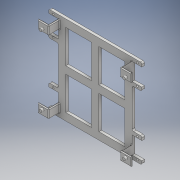
# Autodesk Inventor part: kadlub
Saved by Autodesk Inventor 2018 (Build 220112000, 112)
## iProperties
Created: 2020-10-03
Part Number: kadlub
Material: Ogólny
Document SubType Name: Modeling
Designer: Raven
Density: 1 g/cm^3
Appearance: Domyślna
Author: Raven
Autodesk Inventor part; units mm, degrees
ref_plane "YZ Plane" through (0, 0, 0) normal (1, 0, 0) x (0, 1, 0)
ref_plane "XZ Plane" through (0, 0, 0) normal (0, 1, 0) x (-1, 0, 0)
ref_plane "XY Plane" through (0, 0, 0) normal (0, 0, 1) x (1, 0, 0)
sketch "Szkic1" plane through (0, 0, 0) normal (0, 1, 0) x (-1, 0, 0)
  line L0 (0, 0) -> (50, 0) construction
  line L1 (50, 0) -> (50, -60) construction
  line L2 (50, -60) -> (0, -60) construction
  line L3 (0, -60) -> (0, 0) construction
  line L4 (50, -60) -> (20, -60) construction
  line L5 (20, -60) -> (20, -30) construction
  line L6 (20, -30) -> (50, -30) construction
  line L7 (50, -30) -> (50, -60) construction
  line L8 (20, -30) -> (76.5685, -86.5685) construction
  line L9 (20, -30) -> (100, -30) construction
  line L10 (50, -60) -> (-50, -60)
  line L11 (-50, -60) -> (-50, 60)
  line L12 (-50, 60) -> (50, 60)
  line L13 (50, 60) -> (50, -60)
  dimension "d0" = 50
  dimension "d1" = 60
  dimension "d2" = 30
  dimension "d3" = 30
  dimension "d4" = 80
  dimension "d5" = 45
  dimension "d6" = 100
  dimension "d7" = 120
  constraints: 28 end point, 6 parallel, 4 horizontal, 3 perpendicular, 1 equal length
  measures "d0" distance of L1.end L2.end
  measures "d1" distance of L0.end L1.end
  measures "d2" distance of L5.end L6.end
  measures "d3" distance of L4.end L5.end
  measures "d4" distance of L5.end L8.end
  measures "d5" angle of L8 L9
  measures "d6" distance of L11.end L12.end
  measures "d7" distance of L10.end L11.end
extrude "Wyciągnięcie proste1" add sketch "Szkic1" along normal blind 3.5
sketch "Szkic2" plane through (0, 0, 0) normal (0, -1, 0) x (1, 0, 0)
  line L0 (-50, 60) -> (-50, -60) construction
  line L1 (50, -60) -> (-50, -60) projected
  line L2 (-50, -60) -> (-63.2, -60)
  line L3 (-63.2, -60) -> (-63.2, -55)
  line L4 (-63.2, -55) -> (-50, -55)
  line L5 (-50, -55) -> (-50, -60)
  line L6 (-57.1, -55) -> (-57.1, -56.9) construction
  circle A0 centre (-57.1, -56.9) radius 1.25
  line L7 (-50, -55) -> (-50, -43.2) construction
  line L8 (-50, -60) -> (-50, 60) construction
  line L9 (-50, -43.2) -> (-68.7012, -43.2) construction
  line L10 (-50, -26.4) -> (-63.2, -26.4)
  line L11 (-63.2, -26.4) -> (-63.2, -31.4)
  line L12 (-63.2, -31.4) -> (-50, -31.4)
  line L13 (-50, -31.4) -> (-50, -26.4)
  line L14 (-57.1, -31.4) -> (-57.1, -29.5) construction
  circle A1 centre (-57.1, -29.5) radius 1.25
  line L15 (0, 0) -> (-82.4094, 0) construction
  line L16 (0, -60) -> (0, 60) construction
  line L17 (-50, -60) -> (-50, 60) construction
  line L18 (50, 60) -> (-50, 60)
  line L19 (-50, 60) -> (-63.2, 60)
  line L20 (-63.2, 60) -> (-63.2, 55)
  line L21 (-63.2, 55) -> (-50, 55)
  line L22 (-50, 55) -> (-50, 60)
  line L23 (-57.1, 55) -> (-57.1, 56.9) construction
  circle A2 centre (-57.1, 56.9) radius 1.25
  line L24 (-50, 55) -> (-50, 43.2) construction
  line L25 (-50, 60) -> (-50, -60) construction
  line L26 (-50, 43.2) -> (-68.7012, 43.2) construction
  line L27 (-63.2, 31.4) -> (-50, 31.4)
  line L28 (-50, 26.4) -> (-63.2, 26.4)
  line L29 (-63.2, 26.4) -> (-63.2, 31.4)
  line L30 (-57.1, 31.4) -> (-57.1, 29.5) construction
  circle A3 centre (-57.1, 29.5) radius 1.25
  line L31 (-50, 31.4) -> (-50, 26.4)
  line L32 (50, 60) -> (50, -60) construction
  line L33 (-50, -60) -> (50, -60)
  line L34 (50, -60) -> (63.2, -60)
  line L35 (63.2, -60) -> (63.2, -55)
  line L36 (63.2, -55) -> (50, -55)
  line L37 (50, -55) -> (50, -60)
  line L38 (57.1, -55) -> (57.1, -56.9) construction
  circle A4 centre (57.1, -56.9) radius 1.25
  line L39 (50, -55) -> (50, -43.2) construction
  line L40 (50, -60) -> (50, 60) construction
  line L41 (50, -43.2) -> (68.7012, -43.2) construction
  line L42 (63.2, -31.4) -> (50, -31.4)
  line L43 (50, -26.4) -> (63.2, -26.4)
  line L44 (63.2, -26.4) -> (63.2, -31.4)
  line L45 (57.1, -31.4) -> (57.1, -29.5) construction
  circle A5 centre (57.1, -29.5) radius 1.25
  line L46 (50, -31.4) -> (50, -26.4)
  line L47 (0, 0) -> (82.4094, 0) construction
  line L48 (63.2, 31.4) -> (50, 31.4)
  line L49 (57.1, 31.4) -> (57.1, 29.5) construction
  circle A6 centre (57.1, 29.5) radius 1.25
  line L50 (63.2, 26.4) -> (63.2, 31.4)
  line L51 (50, 31.4) -> (50, 26.4)
  line L52 (50, 26.4) -> (63.2, 26.4)
  line L53 (50, -60) -> (50, 60) construction
  line L54 (50, 60) -> (50, -60) construction
  line L55 (50, 43.2) -> (68.7012, 43.2) construction
  line L56 (63.2, 55) -> (50, 55)
  line L57 (50, 55) -> (50, 43.2) construction
  line L58 (57.1, 55) -> (57.1, 56.9) construction
  circle A7 centre (57.1, 56.9) radius 1.25
  line L59 (50, 60) -> (63.2, 60)
  line L60 (63.2, 60) -> (63.2, 55)
  line L61 (-50, 60) -> (50, 60)
  line L62 (50, 55) -> (50, 60)
  dimension "d41" = 13.2
  dimension "d42" = 5
  dimension "d43" = 1.9
  dimension "d44" = 2.5
  dimension "d45" = 3.1
  dimension "d46" = 11.8
  dimension "d89" = 6.1
  dimension "d90" = 13.2
  dimension "d91" = 13.2
  constraints: 120 end point, 62 symmetric about line, 8 centre point, 8 coincident, 4 point on line, 2 horizontal, 2 perpendicular, 2 vertical, 1 midpoint, 1 parallel, 7 other
  measures "d41" distance of L3.end L4.end
  measures "d42" distance of L2.end L3.end
  measures "d43" distance of L6.start L6.end
  measures "d44" diameter of A0
  measures "d45" distance from line of L2 L6.end
  measures "d46" distance of L4.end L7.end
  measures "d89" distance of L21.start L23.start
  measures "d90" distance of L17.end L19.end
  measures "d91" distance of L21.start L21.end
extrude "Wyciągnięcie proste2" add sketch "Szkic2" against normal blind 3.5
sketch "Szkic3" plane through (0, 0, 0) normal (0, -1, 0) x (1, 0, 0)
  circle A0 centre (57.1, -56.9) radius 1.25 construction
  circle A1 centre (57.1, 29.5) radius 1.25 construction
  circle A2 centre (-57.1, 29.5) radius 1.25 construction
  circle A3 centre (-57.1, -56.9) radius 1.25 construction
  circle A4 centre (-57.1, -29.5) radius 1.25 construction
  circle A5 centre (-57.1, 56.9) radius 1.25 construction
  circle A6 centre (57.1, -29.5) radius 1.25 construction
  circle A7 centre (57.1, 56.9) radius 1.25 construction
  line L0 (-63.2, -60) -> (63.2, -60) construction
  line L1 (63.2, -55) -> (63.2, -60) construction
  line L2 (50, -55) -> (63.2, -55) construction
  line L3 (50, -55) -> (50, -31.4) construction
  line L4 (63.2, -31.4) -> (50, -31.4) construction
  line L5 (63.2, -26.4) -> (63.2, -31.4) construction
  line L6 (50, -26.4) -> (63.2, -26.4) construction
  line L7 (50, -26.4) -> (50, 26.4) construction
  line L8 (63.2, 26.4) -> (50, 26.4) construction
  line L9 (63.2, 31.4) -> (63.2, 26.4) construction
  line L10 (50, 31.4) -> (63.2, 31.4) construction
  line L11 (50, 31.4) -> (50, 55) construction
  line L12 (63.2, 55) -> (50, 55) construction
  line L13 (63.2, 60) -> (63.2, 55) construction
  line L14 (63.2, 60) -> (-63.2, 60) construction
  line L15 (-63.2, 60) -> (-63.2, 55) construction
  line L16 (-63.2, 55) -> (-50, 55) construction
  line L17 (-50, 55) -> (-50, 31.4) construction
  line L18 (-50, 31.4) -> (-63.2, 31.4) construction
  line L19 (-63.2, 31.4) -> (-63.2, 26.4) construction
  line L20 (-63.2, 26.4) -> (-50, 26.4) construction
  line L21 (-50, 26.4) -> (-50, -26.4) construction
  line L22 (-50, -26.4) -> (-63.2, -26.4) construction
  line L23 (-63.2, -26.4) -> (-63.2, -31.4) construction
  line L24 (-63.2, -31.4) -> (-50, -31.4) construction
  line L25 (-50, -31.4) -> (-50, -55) construction
  line L26 (-63.2, -55) -> (-50, -55) construction
  line L27 (-63.2, -60) -> (-63.2, -55) construction
  line L28 (-63.2, -60) -> (63.2, -60) construction
  line L29 (-50, 26.4) -> (-50, -26.4) construction
  line L30 (-50, 60) -> (-50, 50) construction
  line L31 (-50, 55) -> (-50, 31.4) construction
  line L32 (-50, 50) -> (50, 50) construction
  line L33 (50, 31.4) -> (50, 55) construction
  line L34 (45, 60) -> (35, 60) construction
  line L35 (50, -60) -> (50, -50) construction
  line L36 (50, -55) -> (50, -31.4) construction
  line L37 (50, -50) -> (-50, -50) construction
  line L38 (-50, -31.4) -> (-50, -55) construction
  line L39 (-50, -60) -> (-40, -60) construction
  line L40 (-40, -60) -> (-40, 60) construction
  line L41 (0, 60) -> (-5, 60) construction
  line L42 (-5, 60) -> (-5, -60) construction
  line L43 (0, 60) -> (5, 60) construction
  line L44 (5, 60) -> (5, -60) construction
  line L45 (-50, 0) -> (-50, 5) construction
  line L46 (-50, 5) -> (50, 5) construction
  line L47 (50, -26.4) -> (50, 26.4) construction
  line L48 (-50, 0) -> (-50, -5) construction
  line L49 (-50, -5) -> (50, -5) construction
  line L50 (63.2, 60) -> (-63.2, 60) construction
  line L51 (50, 60) -> (40, 60) construction
  line L52 (40, 60) -> (40, -60) construction
  line L53 (5, -5) -> (40, -5)
  line L54 (40, -5) -> (40, -50)
  line L55 (40, -50) -> (5, -50)
  line L56 (5, -50) -> (5, -5)
  line L57 (-5, -5) -> (-40, -5)
  line L58 (-40, -5) -> (-40, -50)
  line L59 (-40, -50) -> (-5, -50)
  line L60 (-5, -50) -> (-5, -5)
  line L61 (-40, 5) -> (-5, 5)
  line L62 (-5, 5) -> (-5, 50)
  line L63 (-5, 50) -> (-40, 50)
  line L64 (-40, 50) -> (-40, 5)
  line L65 (5, 50) -> (40, 50)
  line L66 (40, 50) -> (40, 5)
  line L67 (40, 5) -> (5, 5)
  line L68 (5, 5) -> (5, 50)
  dimension "d96" = 10
  dimension "d98" = 10
  dimension "d99" = 10
  dimension "d100" = 5
  dimension "d101" = 5
  dimension "d102" = 5
  dimension "d103" = 5
  dimension "d104" = 10
  constraints: 66 end point, 31 point on line, 12 perpendicular, 8 parallel, 4 horizontal, 1 midpoint, 3 other
  measures "d96" distance of L30.start L30.end
  measures "d98" distance of L35.start L35.end
  measures "d99" distance of L39.start L39.end
  measures "d100" distance of L41.start L41.end
  measures "d101" distance of L41.start L43.end
  measures "d102" distance of L45.start L45.end
  measures "d103" distance of L45.start L48.end
  measures "d104" distance of L51.start L51.end
extrude "Wyciągnięcie proste3" cut sketch "Szkic3" against normal blind 3.5
fillet "Zaokrąglenie1" radius 2 8 edges at (-63.2, 1.75, -60) (-63.2, 1.75, -26.4) (-63.2, 1.75, 26.4) (-63.2, 1.75, 60) (63.2, 1.75, 60) (63.2, 1.75, 26.4) (63.2, 1.75, -26.4) (63.2, 1.75, -60)
fillet "Zaokrąglenie2" radius 2 4 edges at (50, 1.75, 26.4) (50, 1.75, -26.4) (-50, 1.75, -26.4) (-50, 1.75, 26.4)
sketch "Szkic4" plane through (0, 0, 0) normal (0, -1, 0) x (1, 0, 0)
  line L0 (-50, 55) -> (-50, 31.4) projected
  line L1 (-63.2, 55) -> (-50, 55) construction
  line L2 (-50, 31.4) -> (-63.2, 31.4) construction
  line L3 (-50, 31.4) -> (-50, 55) projected
  line L4 (-50, 55) -> (-48.5, 55)
  line L5 (-48.5, 55) -> (-48.5, 43.2)
  line L6 (-48.5, 43.2) -> (-50, 43.2)
  line L7 (-50, 43.2) -> (-50, 55)
  line L8 (63.2, 55) -> (50, 55) construction
  line L9 (50, 31.4) -> (50, 55) construction
  line L10 (50, 31.4) -> (63.2, 31.4) construction
  line L11 (50, -55) -> (63.2, -55) construction
  line L12 (-63.2, -55) -> (-50, -55) construction
  line L13 (50, 55) -> (48.5, 55)
  line L14 (48.5, 55) -> (48.5, 43.2)
  line L15 (48.5, 43.2) -> (50, 43.2)
  line L16 (50, 43.2) -> (50, 55)
  line L17 (-63.2, -31.4) -> (-50, -31.4) construction
  line L18 (-50, -31.4) -> (-50, -55) construction
  line L19 (-50, -55) -> (-48.5, -55)
  line L20 (-48.5, -55) -> (-48.5, -43.2)
  line L21 (-48.5, -43.2) -> (-50, -43.2)
  line L22 (-50, -43.2) -> (-50, -55)
  line L23 (50, -55) -> (50, -31.4) construction
  line L24 (63.2, -31.4) -> (50, -31.4) construction
  line L25 (50, -55) -> (48.5, -55)
  line L26 (48.5, -55) -> (48.5, -43.2)
  line L27 (48.5, -43.2) -> (50, -43.2)
  line L28 (50, -43.2) -> (50, -55)
  point P0 (0, 0)
  dimension "d64" = 1.5
  dimension "d65" = 11.8
  dimension "d66" = 1.5
  dimension "d67" = 11.8
  dimension "d106" = 1.5
  dimension "d107" = 11.8
  dimension "d108" = 1.5
  dimension "d109" = 11.8
  constraints: 32 end point, 8 parallel, 4 horizontal, 4 perpendicular
  measures "d64" distance of L5.end L6.end
  measures "d65" distance of L4.end L5.end
  measures "d66" distance of L15.end L14.end
  measures "d67" distance of L14.end L13.end
  measures "d106" distance of L12.end L19.end
  measures "d107" distance of L19.end L20.end
  measures "d108" distance of L11.start L25.end
  measures "d109" distance of L25.end L26.end
extrude "Wyciągnięcie proste4" add sketch "Szkic4" along normal blind 13.3
sketch "Szkic5" plane through (0, -13.3, 0) normal (0, -1, 0) x (1, 0, 0)
  line L0 (-50, 55) -> (-50, 43.2) construction
  line L1 (-50, 43.2) -> (-48.5, 43.2) construction
  line L2 (-48.5, 43.2) -> (-48.5, 55) construction
  line L3 (-48.5, 55) -> (-50, 55) construction
  line L4 (50, 55) -> (48.5, 55) construction
  line L5 (48.5, 55) -> (48.5, 43.2) construction
  line L6 (48.5, 43.2) -> (50, 43.2) construction
  line L7 (50, 43.2) -> (50, 55) construction
  line L8 (50, -31.4) -> (48.5, -31.4) construction
  line L9 (48.5, -31.4) -> (48.5, -55) construction
  line L10 (48.5, -55) -> (50, -55) construction
  line L11 (50, -55) -> (50, -31.4) construction
  line L12 (-48.5, -31.4) -> (-50, -31.4) construction
  line L13 (-50, -31.4) -> (-50, -55) construction
  line L14 (-50, -55) -> (-48.5, -55) construction
  line L15 (-48.5, -55) -> (-48.5, -31.4) construction
  line L16 (63.2, 55) -> (50, 55) construction
  line L17 (-63.2, 55) -> (-50, 55) construction
  line L18 (-48.5, 55) -> (-63.2, 55)
  line L19 (-63.2, 55) -> (-63.2, 43.2)
  line L20 (-63.2, 43.2) -> (-48.5, 43.2)
  line L21 (-48.5, 43.2) -> (-48.5, 55)
  line L22 (48.5, 55) -> (63.2, 55)
  line L23 (63.2, 55) -> (63.2, 43.2)
  line L24 (63.2, 43.2) -> (48.5, 43.2)
  line L25 (48.5, 43.2) -> (48.5, 55)
  line L26 (50, -55) -> (63.2, -55) construction
  line L27 (48.5, -55) -> (50, -55) construction
  line L28 (50, -55) -> (50, -43.2) construction
  line L29 (50, -43.2) -> (48.5, -43.2) construction
  line L30 (48.5, -43.2) -> (48.5, -55) construction
  line L31 (-63.2, -55) -> (-50, -55) construction
  line L32 (-50, -55) -> (-48.5, -55) construction
  line L33 (-48.5, -55) -> (-48.5, -43.2) construction
  line L34 (-48.5, -43.2) -> (-50, -43.2) construction
  line L35 (-50, -43.2) -> (-50, -55) construction
  line L36 (-48.5, -55) -> (-63.2, -55)
  line L37 (-63.2, -55) -> (-63.2, -43.2)
  line L38 (-63.2, -43.2) -> (-48.5, -43.2)
  line L39 (-48.5, -43.2) -> (-48.5, -55)
  line L40 (48.5, -55) -> (63.2, -55)
  line L41 (63.2, -55) -> (63.2, -43.2)
  line L42 (63.2, -43.2) -> (48.5, -43.2)
  line L43 (48.5, -43.2) -> (48.5, -55)
  point P0 (0, 0)
  constraints: 32 end point, 8 parallel, 4 horizontal, 4 perpendicular, 1 point on line
extrude "Wyciągnięcie proste5" add sketch "Szkic5" along normal blind 1.5
sketch "Szkic6" plane through (0, -14.8, 0) normal (0, -1, 0) x (1, 0, 0)
  line L0 (-50, 55) -> (-50, 43.2) construction
  line L1 (-48.5, 55) -> (-63.2, 55) construction
  line L2 (-48.5, 55) -> (-63.2, 55) construction
  line L3 (-63.2, 55) -> (-63.2, 31.4) construction
  line L4 (-63.2, 31.4) -> (-48.5, 31.4) construction
  line L5 (-48.5, 31.4) -> (-48.5, 55) construction
  line L6 (50, 43.2) -> (50, 55) construction
  line L7 (63.2, 55) -> (48.5, 55) construction
  line L8 (48.5, 55) -> (48.5, 31.4) construction
  line L9 (48.5, 31.4) -> (63.2, 31.4) construction
  line L10 (63.2, 31.4) -> (63.2, 55) construction
  line L11 (50, -55) -> (50, 55) construction
  line L12 (63.2, -31.4) -> (48.5, -31.4) construction
  line L13 (48.5, -31.4) -> (48.5, -55) construction
  line L14 (48.5, -55) -> (63.2, -55) construction
  line L15 (63.2, -55) -> (63.2, -31.4) construction
  line L16 (-50, 55) -> (-50, -55) construction
  line L17 (-48.5, -31.4) -> (-63.2, -31.4) construction
  line L18 (-63.2, -31.4) -> (-63.2, -55) construction
  line L19 (-63.2, -55) -> (-48.5, -55) construction
  line L20 (-48.5, -55) -> (-48.5, -31.4) construction
  line L21 (-50, 55) -> (-63.2, 55) construction
  line L22 (-50, 55) -> (-63.2, 55) construction
  circle A0 centre (-56.6, 47.4) radius 1.95
  line L23 (63.2, 55) -> (50, 55) construction
  circle A1 centre (56.6, 47.4) radius 1.95
  line L24 (63.2, -55) -> (50, -55) construction
  line L25 (-63.2, -55) -> (-50, -55) construction
  circle A2 centre (56.6, -47.4) radius 1.95
  circle A3 centre (-56.6, -47.4) radius 1.95
  line L26 (63.2, -31.4) -> (50, -31.4) construction
  line L27 (-50, -31.4) -> (-63.2, -31.4) construction
  line L28 (-50, 55) -> (-63.2, 55) projected
  line L29 (50, -55) -> (63.2, -55) construction
  point P0 (0, 0)
  dimension "d79" = 3.9
  dimension "d81" = 3.9
  dimension "d84" = 3.9
  dimension "d85" = 3.9
  constraints: 4 centre point, 2 end point, 1 perpendicular
  measures "d79" diameter of A0
  measures "d81" diameter of A1
  measures "d84" diameter of A2
  measures "d85" diameter of A3
extrude "Wyciągnięcie proste6" add sketch "Szkic6" along normal blind 3
fillet "Zaokrąglenie4" radius 1 36 edges at (-48.5, 0, 49.1) (-49.25, 0, 43.2) (-48.5, -7.4, 43.2) (-48.5, -7.4, 55) (-49.25, 0, 55) (48.5, 0, 49.1) (48.5, -7.4, 43.2) (49.25, 0, 43.2) (48.5, -7.4, 55) (49.25, 0, 55) (48.5, 0, -49.1) (48.5, -7.4, -55) (49.25, 0, -55) (-48.5, -7.4, -55) (-49.25, 0, -55) (-48.5, 0, -49.1) (-48.5, -7.4, -43.2) (-49.25, 0, -43.2) (-55.85, -14.8, -43.2) (-63.2, -14.8, -49.1) (-55.85, -14.8, -55) (-55.85, -14.8, 55) (-48.5, -14.8, 49.1) (-55.85, -14.8, 43.2) (-63.2, -14.8, 49.1) (48.5, -14.8, 49.1) (55.85, -14.8, 55) (63.2, -14.8, 49.1) (55.85, -14.8, 43.2) (55.85, -14.8, -55) (49.25, 0, -43.2) (48.5, -7.4, -43.2) (55.85, -14.8, -43.2) (48.5, -14.8, -49.1) (63.2, -14.8, -49.1) (-48.5, -14.8, -49.1)
equation "\"d81\" = d79"
equation "\"d84\" = d79"
equation "\"d85\" = d79"
